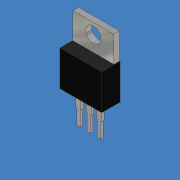
# Autodesk Inventor part: Fet
Saved by Autodesk Inventor 2011 SP1 (Build 150282100, 282)
## iProperties
Shininess: 64.0
Length Units: 11272
Angle Units: 11279
Time Units: 11290
Mass Units: 11286
Length Display Precision: 3
Angle Display Precision: 2
Compacted: True
Part Number: Fet
Document SubType Name: Modeling
Created: 2007-01-15
Designer: uidk0133
Density: 1 g/cm^3
Density: 0.0
Volumn: 0.0
Area: 0.0
PropertySet Name: Model Information
Control State: 0
Master: False
Checked Out: False
Author: uidk0133
Autodesk Inventor part; units mm, degrees
ref_plane "YZ Plane" through (0, 0, 0) normal (1, 0, 0) x (0, 1, 0)
ref_plane "XZ Plane" through (0, 0, 0) normal (0, 1, 0) x (-1, 0, 0)
ref_plane "XY Plane" through (0, 0, 0) normal (0, 0, 1) x (1, 0, 0)
sketch "Sketch1" plane through (0, 0, 0) normal (0, 0, 1) x (1, 0, 0)
  line L0 (-5.08, 8.636) -> (5.08, 8.636)
  line L1 (5.08, 8.636) -> (5.08, 0)
  line L2 (5.08, 0) -> (-5.08, 0)
  line L3 (-5.08, 0) -> (-5.08, 8.636)
  point P0 (0, 0)
  point P1 (0, 0)
  dimension "d0" = 10.16
  dimension "d1" = 8.636
  constraints: 8 end point, 2 parallel, 1 coincident, 1 horizontal, 1 midpoint, 1 perpendicular, 1 other
  measures "d0" distance of L0.start L0.end
  measures "d1" distance of L0.end L1.end
extrude "Extrusion1" add sketch "Sketch1" along normal blind 4.4704
sketch "Sketch2" plane through (-5.08, 8.636, 0) normal (0, 1, 0) x (1, 0, 0)
  line L0 (0.0889, -1.397) -> (10.0711, -1.397)
  line L1 (10.0711, -1.397) -> (10.0711, 0)
  line L2 (10.0711, 0) -> (0.0889, 0)
  line L3 (0.0889, 0) -> (0.0889, -1.397)
  line L4 (0, 0) -> (10.16, 0) projected
  point P0 (5.08, 0)
  dimension "d7" = 1.397
  dimension "d8" = 9.9822
  constraints: 8 end point, 2 midpoint, 2 parallel, 1 horizontal, 1 perpendicular
  measures "d7" distance of L2.end L0.start
  measures "d8" distance of L0.start L0.end
extrude "Extrusion2" add sketch "Sketch2" along normal blind 6.35
sketch "Sketch3" plane through (-4.9911, 8.636, 1.397) normal (0, 0, 1) x (1, 0, 0)
  line L0 (9.9822, 6.35) -> (0, 6.35) projected
  line L1 (9.9822, 0) -> (9.9822, 6.35) projected
  line L2 (4.9911, 6.35) -> (4.9911, 1.588) construction
  point P0 (4.9911, 3.81)
  dimension "d9" = 2.54
  constraints: 2 end point, 1 midpoint, 1 parallel, 1 point on line
  measures "d9" distance from line of L0 point (4.991, 3.81)
hole "Hole1" at (0, 12.446, 1.397) direction (0, 0, -1) diameter 3.683 end through all
sketch "Sketch4" plane through (-5.08, 0, 0) normal (0, -1, 0) x (1, 0, 0)
  line L0 (0, 0) -> (0, 4.4704) projected
  line L1 (10.16, 0) -> (10.16, 4.4704) projected
  line L2 (0, 2.2352) -> (10.16, 2.2352) construction
  line L3 (1.905, 2.5273) -> (3.175, 2.5273)
  line L4 (3.175, 2.5273) -> (3.175, 1.9431)
  line L5 (3.175, 1.9431) -> (1.905, 1.9431)
  line L6 (1.905, 1.9431) -> (1.905, 2.5273)
  point P0 (1.905, 2.2352)
  dimension "d17" = 0.5842
  dimension "d18" = 1.27
  dimension "d19" = 1.905
  constraints: 10 end point, 3 midpoint, 2 parallel, 1 horizontal, 1 perpendicular, 1 point on line
  measures "d17" distance of L3.end L4.end
  measures "d18" distance of L4.end L5.end
  measures "d19" distance from line of L0 L3.start
extrude "Extrusion3" add sketch "Sketch4" along normal blind 3.81
sketch "Sketch5" plane through (-5.08, -3.81, 0) normal (0, -1, 0) x (1, 0, 0)
  line L0 (1.905, 2.5273) -> (3.175, 2.5273) projected
  line L1 (3.175, 1.9431) -> (1.905, 1.9431) projected
  line L2 (2.1336, 2.5273) -> (2.9464, 2.5273)
  line L3 (2.9464, 2.5273) -> (2.9464, 1.9431)
  line L4 (2.9464, 1.9431) -> (2.1336, 1.9431)
  line L5 (2.1336, 1.9431) -> (2.1336, 2.5273)
  point P0 (2.54, 1.9431)
  dimension "d22" = 0.8128
  constraints: 8 end point, 2 midpoint, 2 parallel, 2 point on line, 1 horizontal, 1 perpendicular
  measures "d22" distance between parallel lines of L3 L5
extrude "Extrusion4" add sketch "Sketch5" along normal blind 3.81
pattern_linear "Rectangular Pattern1" count 3 spacing 2.54 along (1, 0, 0) of "Extrusion4", "Extrusion3"
body "Solid1"
